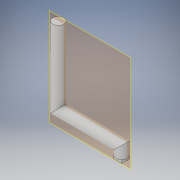
# Autodesk Inventor part: handle
Saved by Autodesk Inventor 2019 (Build 230136000, 136)
## iProperties
Created: 2020-02-24
Part Number: handle
Material: Generic
Document SubType Name: Modeling
Designer: Jeff
Density: 1 g/cm^3
Appearance: Default
Author: Jeff
Autodesk Inventor part; units mm, degrees
ref_plane "YZ Plane" through (0, 0, 0) normal (1, 0, 0) x (0, 1, 0)
ref_plane "XZ Plane" through (0, 0, 0) normal (0, 1, 0) x (-1, 0, 0)
sketch "Sketch1" plane through (0, 0, 0) normal (0, 1, 0) x (-1, 0, 0)
  line L0 (-4.625, 4.625) -> (4.625, 4.625)
  line L1 (4.625, 4.625) -> (4.625, -4.625)
  line L2 (4.625, -4.625) -> (-4.625, -4.625)
  line L3 (-4.625, -4.625) -> (-4.625, 4.625)
  point P0 (0, 0)
  point P1 (4.625, 0)
  point P2 (0, -4.625)
  dimension "d0" = 9.25
  constraints: 8 end point, 2 midpoint, 2 parallel, 2 perpendicular, 1 horizontal, 1 horizontal alignment, 1 vertical alignment
  measures "d0" distance of L0.end L1.end
extrude "Extrusion1" add sketch "Sketch1" along normal blind 4
sketch "Sketch2" plane through (0, 4, 0) normal (0, 1, 0) x (1, 0, 0)
  line L0 (4.625, 4.625) -> (-4.625, 4.625) projected
  circle A0 centre (0, 0) radius 6.5407
  constraints: 1 coincident, 3 other
sketch "Sketch3" plane through (0, 0, 0) normal (0, 0, 1) x (1, 0, 0)
  line L0 (-4.625, 4) -> (4.625, 4) projected
  line L1 (0, 4) -> (0, 14)
  line L2 (0, 14) -> (-75, 14)
  line L3 (-75, 14) -> (-75, 104)
  point P0 (0, 0)
  dimension "d3" = 10
  dimension "d4" = 75
  dimension "d5" = 90
  constraints: 6 end point, 2 perpendicular, 1 midpoint, 1 vertical
  measures "d3" distance of L1.start L1.end
  measures "d4" distance of L1.end L2.end
  measures "d5" distance of L2.end L3.end
sweep "Sweep1" add profiles "Sketch2" path "Sketch3" path curves L1 L2 L3
body "Solid1"
